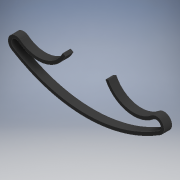
# Autodesk Inventor part: 脚ゴム2
Saved by Autodesk Inventor 2020 (Build 240168000, 168)
## iProperties
Created: 2019-09-03
Part Number: 脚ゴム2
Material: ゴム、シリコーン
Document SubType Name: Modeling
Designer: 雪村
Mass: 2.43996 g
Surface Area: 27.5274 cm^2
Volume: 1.95196 cm^3
Density: 1.25 g/cm^3
Appearance: ゴム - 黒
Author: 雪村
Autodesk Inventor part; units mm, degrees
ref_plane "YZ Plane" through (0, 0, 0) normal (1, 0, 0) x (0, 1, 0)
ref_plane "XZ Plane" through (0, 0, 0) normal (0, 1, 0) x (-1, 0, 0)
ref_plane "XY Plane" through (0, 0, 0) normal (0, 0, 1) x (1, 0, 0)
sketch "スケッチ1" plane through (0, 0, 0) normal (0, 0, 1) x (1, 0, 0)
  spline S0 degree 4 poles (-46.7287, -62.3958) (-46.4075, -62.5897) (-45.9582, -62.8581) (-45.3809, -63.1982) (-44.6755, -63.6062) (-44.164, -63.8983) (-43.6533, -64.1863) (-43.1431, -64.4703) (-42.6335, -64.7504) (-42.1242, -65.0266) (-41.6152, -65.299) (-41.1064, -65.5676) (-40.5978, -65.8326) (-40.0892, -66.0938) (-39.5807, -66.3514) (-39.072, -66.6054) (-38.5633, -66.8559) (-38.0543, -67.1029) (-37.5452, -67.3463) (-37.0357, -67.5863) (-36.526, -67.8228) (-36.0159, -68.0558) (-35.5054, -68.2855) (-34.9944, -68.5118) (-34.483, -68.7346) (-33.9711, -68.9542) (-33.4587, -69.1703) (-32.9457, -69.3831) (-32.4322, -69.5925) (-31.9181, -69.7986) (-31.4034, -70.0014) (-30.8881, -70.2009) (-30.3721, -70.397) (-29.8555, -70.5898) (-29.3383, -70.7793) (-28.8203, -70.9655) (-28.3017, -71.1484) (-27.7825, -71.3279) (-27.2625, -71.5041) (-26.7419, -71.6771) (-26.2205, -71.8467) (-25.6985, -72.0129) (-25.1758, -72.1759) (-24.6524, -72.3355) (-24.1283, -72.4918) (-23.6035, -72.6447) (-23.078, -72.7943) (-22.5519, -72.9406) (-22.0251, -73.0835) (-21.4976, -73.2231) (-20.9695, -73.3593) (-20.4407, -73.4921) (-19.9113, -73.6216) (-19.3812, -73.7477) (-18.8505, -73.8704) (-18.3193, -73.9897) (-17.7874, -74.1057) (-17.2549, -74.2182) (-16.7219, -74.3274) (-16.1883, -74.4332) (-15.6541, -74.5355) (-15.1195, -74.6344) (-14.5843, -74.7299) (-14.0486, -74.822) (-13.5124, -74.9107) (-12.9757, -74.9959) (-12.4386, -75.0776) (-11.901, -75.156) (-11.363, -75.2309) (-10.8247, -75.3023) (-10.2859, -75.3703) (-9.7467, -75.4348) (-9.2072, -75.4958) (-8.6674, -75.5534) (-8.1272, -75.6075) (-7.5868, -75.6581) (-7.046, -75.7053) (-6.5051, -75.749) (-5.9638, -75.7892) (-5.4224, -75.8259) (-4.8807, -75.8591) (-4.3389, -75.8888) (-3.7969, -75.915) (-3.2547, -75.9378) (-2.7125, -75.957) (-2.1701, -75.9728) (-1.6276, -75.985) (-1.0851, -75.9938) (-0.5426, -75.999) (0, -76.0008) (0.5426, -75.999) (1.0851, -75.9938) (1.6276, -75.985) (2.1701, -75.9728) (2.7124, -75.957) (3.2547, -75.9378) (3.7969, -75.915) (4.3388, -75.8888) (4.8807, -75.8591) (5.4223, -75.8259) (5.9638, -75.7892) (6.505, -75.749) (7.046, -75.7053) (7.5867, -75.6582) (8.1271, -75.6075) (8.6672, -75.5534) (9.207, -75.4958) (9.7465, -75.4348) (10.2856, -75.3703) (10.8243, -75.3023) (11.3626, -75.2309) (11.9005, -75.156) (12.4379, -75.0777) (12.9749, -74.9959) (13.5114, -74.9108) (14.0474, -74.8221) (14.5829, -74.7301) (15.1179, -74.6346) (15.6524, -74.5357) (16.1862, -74.4334) (16.7195, -74.3277) (17.2522, -74.2186) (17.7843, -74.1061) (18.3158, -73.9902) (18.8466, -73.871) (19.3768, -73.7483) (19.9062, -73.6223) (20.435, -73.493) (20.9632, -73.3602) (21.4905, -73.2242) (22.0172, -73.0848) (22.5431, -72.9421) (23.0683, -72.796) (23.5927, -72.6466) (24.1163, -72.4939) (24.6392, -72.3379) (25.1612, -72.1786) (25.6825, -72.0161) (26.2029, -71.8502) (26.7225, -71.681) (27.2413, -71.5086) (27.7593, -71.3329) (28.2764, -71.154) (28.7926, -70.9718) (29.308, -70.7863) (29.8225, -70.5976) (30.3362, -70.4057) (30.849, -70.2105) (31.3609, -70.0121) (31.8719, -69.8105) (32.3821, -69.6057) (32.8914, -69.3976) (33.3998, -69.1863) (33.9073, -68.9719) (34.414, -68.7542) (34.9198, -68.5333) (35.4247, -68.3093) (35.9288, -68.082) (36.432, -67.8516) (36.9344, -67.6179) (37.4359, -67.381) (37.9366, -67.141) (38.4364, -66.8977) (38.9355, -66.6513) (39.4337, -66.4016) (39.9312, -66.1488) (40.4279, -65.8927) (40.9238, -65.6334) (41.419, -65.3709) (41.9135, -65.1051) (42.4073, -64.8361) (42.9004, -64.5639) (43.3928, -64.2884) (43.8846, -64.0096) (44.3758, -63.7275) (44.8664, -63.4421) (45.3565, -63.1534) (46.0301, -62.7516) (46.5798, -62.4176) (47.0065, -62.1545) (47.3109, -61.9649) knots 0 0 0 0 0 0.014459 0.020221 0.025968 0.031703 0.037425 0.043135 0.048834 0.054523 0.060202 0.065871 0.071532 0.077184 0.082829 0.088465 0.094095 0.099718 0.105334 0.110945 0.11655 0.122149 0.127744 0.133333 0.138918 0.144499 0.150076 0.155648 0.161217 0.166783 0.172345 0.177904 0.183461 0.189014 0.194565 0.200113 0.205659 0.211203 0.216745 0.222285 0.227822 0.233359 0.238893 0.244426 0.249957 0.255487 0.261016 0.266543 0.272069 0.277594 0.283118 0.288641 0.294163 0.299685 0.305205 0.310725 0.316243 0.321762 0.327279 0.332796 0.338313 0.343828 0.349344 0.354859 0.360373 0.365887 0.371401 0.376914 0.382427 0.38794 0.393452 0.398964 0.404476 0.409988 0.415499 0.421011 0.426522 0.432033 0.437544 0.443054 0.448565 0.454075 0.459586 0.465096 0.470606 0.476117 0.481627 0.487137 0.492647 0.498157 0.503667 0.509177 0.514688 0.520198 0.525708 0.531218 0.536729 0.542239 0.54775 0.553261 0.558771 0.564282 0.569793 0.575304 0.580816 0.586327 0.591839 0.597351 0.602863 0.608375 0.613888 0.6194 0.624913 0.630427 0.63594 0.641454 0.646969 0.652483 0.657998 0.663514 0.66903 0.674546 0.680063 0.68558 0.691098 0.696617 0.702136 0.707656 0.713176 0.718697 0.724219 0.729741 0.735265 0.740789 0.746314 0.75184 0.757367 0.762895 0.768424 0.773955 0.779486 0.785019 0.790553 0.796089 0.801626 0.807165 0.812705 0.818247 0.82379 0.829336 0.834883 0.840433 0.845984 0.851538 0.857094 0.862653 0.868214 0.873778 0.879345 0.884914 0.890487 0.896063 0.901642 0.907224 0.912811 0.918401 0.923995 0.929593 0.935196 0.940803 0.946414 0.952031 0.957653 0.96328 0.968913 0.974552 0.980196 0.985847 1 1 1 1 1
  arc A0 (-43.3371, -57.4602) -> (-46.7287, -62.3958) centre (-45.1853, -59.8233) ccw
  arc A1 (-43.3371, -57.4602) -> (-12.9977, -50.3865) centre (-31.0158, -41.7063) ccw
  arc A2 (12.8817, -50.3865) -> (43.8031, -57.1163) centre (30.9439, -41.7983) ccw
  arc A3 (47.3109, -61.9649) -> (43.8031, -57.1163) centre (45.732, -59.414) ccw
  arc A4 (-42.105, -55.8848) -> (-14.7995, -49.5185) centre (-31.0158, -41.7063) ccw
  arc A5 (-42.105, -55.8848) -> (-47.7601, -64.1093) centre (-45.1853, -59.8233) ccw
  arc A6 (48.3661, -63.6639) -> (42.5172, -55.5845) centre (45.732, -59.414) ccw
  arc A7 (14.6879, -49.5277) -> (42.5172, -55.5845) centre (30.9439, -41.7983) ccw
  line L0 (-12.9977, -50.3865) -> (-14.7995, -49.5185)
  line L1 (12.8817, -50.3865) -> (14.6879, -49.5277)
  spline S1 degree 5 poles (-47.7621, -64.1081) (-39.0585, -69.3622) (-29.7722, -73.6606) (-19.8779, -76.6074) (0.4344, -79.4943) (20.7174, -76.4) (30.5408, -73.3687) (39.7688, -69.0175) (48.3682, -63.6626) knots 0 0 0 0 0 0 0.500897 0.500897 0.500897 1 1 1 1 1 1
  point P0 (0, 0)
  point P1 (0, 0)
  dimension "d0" = 2
  constraints: 16 point on circle, 8 centre point, 4 end point, 2 concentric, 2 line through centre, 15 other
  measures "d0" radial gap between concentric circles of A1 A4
extrude "押し出し1" add sketch "スケッチ1" along normal blind 5
